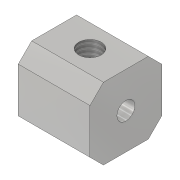
# Autodesk Inventor part: Aluminium_Block_Motor
Saved by Autodesk Inventor 2018.3 (Build 223284000, 284)
## iProperties
Created: 2019-03-20
Part Number: Aluminium_Block_Motor
Material: Generisch
Document SubType Name: Modeling
Designer: rhoch
Density: 1 g/cm^3
Appearance: Vorgabe
Author: rhoch
Autodesk Inventor part; units mm, degrees
ref_plane "YZ Plane" through (0, 0, 0) normal (1, 0, 0) x (0, 1, 0)
ref_plane "XZ Plane" through (0, 0, 0) normal (0, 1, 0) x (-1, 0, 0)
ref_plane "XY Plane" through (0, 0, 0) normal (0, 0, 1) x (1, 0, 0)
sketch "Skizze2" plane through (0, 0, 0) normal (1, 0, 0) x (0, 1, 0)
  line L0 (4, 4) -> (-4, 4)
  line L1 (-4, 4) -> (-4, -4)
  line L2 (-4, -4) -> (4, -4)
  line L3 (4, -4) -> (4, 4)
  point P0 (0, 0)
  point P1 (0, 0)
  dimension "d7" = 8
  dimension "d8" = 8
  dimension "d9" = 4
  dimension "d10" = 4
  constraints: 8 end point, 2 parallel, 1 coincident, 1 horizontal, 1 perpendicular
  measures "d7" distance between parallel lines of L1 L3
  measures "d8" distance between parallel lines of L2 L0
  measures "d9" distance from line of point (0, 0) L2
  measures "d10" distance from line of L1 point (0, 0)
extrude "Extrusion1" add sketch "Skizze2" along normal blind 8
chamfer "Fase1" distance 1.5 angle 45 4 edges at (4, 4, 4) (4, 4, -4) (4, -4, 4) (4, -4, -4)
hole "Bohrung1" at (0, 0, 0) direction (1, 0, 0) diameter 2 end through all counterbore diameter 4 counterbore depth 1
sketch "Skizze3" plane through (0, -2.5, -4) normal (0, 0, -1) x (-1, 0, 0)
  line L0 (0, 0) -> (0, 5) projected
  line L1 (-8, -1.5) -> (0, -1.5) projected
  point P0 (0, 2.5)
  point P1 (-4, 2.5)
  dimension "d23" = 4
  dimension "d24" = 4
  measures "d23" distance from line of L0 point (-4, 2.5)
  measures "d24" distance from line of L1 point (-4, 2.5)
hole "Bohrung2" at (4, 0, -4) direction (0, 0, 1) diameter 2.5 end through all
thread "Gewinde1" size "M3x0.5" class "6H" standard "ANSI Metric M Profile" full length
